Autodesk Inventor part; units mm, degrees
(part 2 of 2)
  measures "d102" distance from line of L722 point (11.407, 32.366)
  measures "d103" distance of point (11.407, 32.366) L722.start
  measures "d104" distance from line of point (37.447, 72.366) L723
  measures "d105" horizontal distance of A1.centre point (49.32, 36.16)
  measures "d106" horizontal distance of point (49.32, 36.16) A1.centre
extrude "Extrusion7" cut sketch "Sketch11" against normal blind 10 contours L0 L1 L2 L3 | L6 L7 L8 L9 | L10 L11 L12 L13 | L14 L15 L16 L17 | L18 L19 L20 L21 | L22 L23 L24 L25 | A0 L365 L362 L363 | A0 L312 L313 L310 L311 | A0 L144 L145 L142 L143 | L62 L63 L64 L65 | L66 L67 L68 L69 | L70 L71 L72 L73 | L74 L75 L76 L77 | L78 L79 L80 L81 | L82 L83 L84 L85 | L122 L123 L124 L125 | L126 L127 L128 L129 | L130 L131 L132 L133 | L134 L135 L136 L137 | L138 L139 L140 L141 | L182 L183 L184 L185 | L186 L187 L188 L189 | L190 L191 L192 L193 | L194 L195 L196 L197 | L198 L199 L200 L201 | L242 L243 L244 L245 | L246 L247 L248 L249 | L250 L251 L252 L253 | L254 L255 L256 L257 | L302 L303 L304 L305 | L306 L307 L308 L309
sketch "Sketch12" plane through (0, 2, 0) normal (0, 1, 0) x (1, 0, 0)
  line L0 (37.4067, 37.3658) -> (39.4067, 37.3658)
  line L1 (39.4067, 37.3658) -> (39.4067, 39.3658)
  line L2 (39.4067, 39.3658) -> (37.4067, 39.3658)
  line L3 (37.4067, 39.3658) -> (37.4067, 37.3658)
  line L4 (35.4067, 37.3658) -> (33.4067, 37.3658) projected
  line L5 (37.4067, 42.8658) -> (39.4067, 42.8658)
  line L6 (39.4067, 42.8658) -> (39.4067, 44.8658)
  line L7 (39.4067, 44.8658) -> (37.4067, 44.8658)
  line L8 (37.4067, 44.8658) -> (37.4067, 42.8658)
  line L9 (37.4067, 48.3658) -> (39.4067, 48.3658)
  line L10 (39.4067, 48.3658) -> (39.4067, 50.3658)
  line L11 (39.4067, 50.3658) -> (37.4067, 50.3658)
  line L12 (37.4067, 50.3658) -> (37.4067, 48.3658)
  line L13 (37.4067, 53.8658) -> (39.4067, 53.8658)
  line L14 (39.4067, 53.8658) -> (39.4067, 55.8658)
  line L15 (39.4067, 55.8658) -> (37.4067, 55.8658)
  line L16 (37.4067, 55.8658) -> (37.4067, 53.8658)
  line L17 (37.4067, 59.3658) -> (39.4067, 59.3658)
  line L18 (39.4067, 59.3658) -> (39.4067, 61.3658)
  line L19 (39.4067, 61.3658) -> (37.4067, 61.3658)
  line L20 (37.4067, 61.3658) -> (37.4067, 59.3658)
  line L21 (37.4067, 64.8658) -> (39.4067, 64.8658)
  line L22 (39.4067, 64.8658) -> (39.4067, 66.8658)
  line L23 (39.4067, 66.8658) -> (37.4067, 66.8658)
  line L24 (37.4067, 66.8658) -> (37.4067, 64.8658)
  line L25 (37.4067, 70.3658) -> (39.4067, 70.3658)
  line L26 (39.4067, 70.3658) -> (39.4067, 72.3658)
  line L27 (39.4067, 72.3658) -> (37.4067, 72.3658)
  line L28 (37.4067, 72.3658) -> (37.4067, 70.3658)
  line L29 (41.4067, 37.3658) -> (43.4067, 37.3658)
  line L30 (43.4067, 37.3658) -> (43.4067, 39.3658)
  line L31 (43.4067, 39.3658) -> (41.4067, 39.3658)
  line L32 (41.4067, 39.3658) -> (41.4067, 37.3658)
  line L33 (41.4067, 42.8658) -> (43.4067, 42.8658)
  line L34 (43.4067, 42.8658) -> (43.4067, 44.8658)
  line L35 (43.4067, 44.8658) -> (41.4067, 44.8658)
  line L36 (41.4067, 44.8658) -> (41.4067, 42.8658)
  line L37 (41.4067, 48.3658) -> (43.4067, 48.3658)
  line L38 (43.4067, 48.3658) -> (43.4067, 50.3658)
  line L39 (43.4067, 50.3658) -> (41.4067, 50.3658)
  line L40 (41.4067, 50.3658) -> (41.4067, 48.3658)
  line L41 (41.4067, 53.8658) -> (43.4067, 53.8658)
  line L42 (43.4067, 53.8658) -> (43.4067, 55.8658)
  line L43 (43.4067, 55.8658) -> (41.4067, 55.8658)
  line L44 (41.4067, 55.8658) -> (41.4067, 53.8658)
  line L45 (41.4067, 59.3658) -> (43.4067, 59.3658)
  line L46 (43.4067, 59.3658) -> (43.4067, 61.3658)
  line L47 (43.4067, 61.3658) -> (41.4067, 61.3658)
  line L48 (41.4067, 61.3658) -> (41.4067, 59.3658)
  line L49 (41.4067, 64.8658) -> (43.4067, 64.8658)
  line L50 (43.4067, 64.8658) -> (43.4067, 66.8658)
  line L51 (43.4067, 66.8658) -> (41.4067, 66.8658)
  line L52 (41.4067, 66.8658) -> (41.4067, 64.8658)
  line L53 (41.4067, 70.3658) -> (43.4067, 70.3658)
  line L54 (43.4067, 70.3658) -> (43.4067, 72.3658)
  line L55 (43.4067, 72.3658) -> (41.4067, 72.3658)
  line L56 (41.4067, 72.3658) -> (41.4067, 70.3658)
  line L57 (45.4067, 37.3658) -> (47.4067, 37.3658)
  line L58 (47.4067, 37.3658) -> (47.4067, 39.3658)
  line L59 (47.4067, 39.3658) -> (45.4067, 39.3658)
  line L60 (45.4067, 39.3658) -> (45.4067, 37.3658)
  line L61 (45.4067, 42.8658) -> (47.4067, 42.8658)
  line L62 (47.4067, 42.8658) -> (47.4067, 44.8658)
  line L63 (47.4067, 44.8658) -> (45.4067, 44.8658)
  line L64 (45.4067, 44.8658) -> (45.4067, 42.8658)
  line L65 (45.4067, 48.3658) -> (47.4067, 48.3658)
  line L66 (47.4067, 48.3658) -> (47.4067, 50.3658)
  line L67 (47.4067, 50.3658) -> (45.4067, 50.3658)
  line L68 (45.4067, 50.3658) -> (45.4067, 48.3658)
  line L69 (45.4067, 53.8658) -> (47.4067, 53.8658)
  line L70 (47.4067, 53.8658) -> (47.4067, 55.8658)
  line L71 (47.4067, 55.8658) -> (45.4067, 55.8658)
  line L72 (45.4067, 55.8658) -> (45.4067, 53.8658)
  line L73 (45.4067, 59.3658) -> (47.4067, 59.3658)
  line L74 (47.4067, 59.3658) -> (47.4067, 61.3658)
  line L75 (47.4067, 61.3658) -> (45.4067, 61.3658)
  line L76 (45.4067, 61.3658) -> (45.4067, 59.3658)
  line L77 (45.4067, 64.8658) -> (47.4067, 64.8658)
  line L78 (47.4067, 64.8658) -> (47.4067, 66.8658)
  line L79 (47.4067, 66.8658) -> (45.4067, 66.8658)
  line L80 (45.4067, 66.8658) -> (45.4067, 64.8658)
  line L81 (45.4067, 70.3658) -> (47.4067, 70.3658)
  line L82 (47.4067, 70.3658) -> (47.4067, 72.3658)
  line L83 (47.4067, 72.3658) -> (45.4067, 72.3658)
  line L84 (45.4067, 72.3658) -> (45.4067, 70.3658)
  line L85 (49.4067, 37.3658) -> (51.4067, 37.3658)
  line L86 (51.4067, 37.3658) -> (51.4067, 39.3658)
  line L87 (51.4067, 39.3658) -> (49.4067, 39.3658)
  line L88 (49.4067, 39.3658) -> (49.4067, 37.3658)
  line L89 (49.4067, 42.8658) -> (51.4067, 42.8658)
  line L90 (51.4067, 42.8658) -> (51.4067, 44.8658)
  line L91 (51.4067, 44.8658) -> (49.4067, 44.8658)
  line L92 (49.4067, 44.8658) -> (49.4067, 42.8658)
  line L93 (49.4067, 48.3658) -> (51.4067, 48.3658)
  line L94 (51.4067, 48.3658) -> (51.4067, 50.3658)
  line L95 (51.4067, 50.3658) -> (49.4067, 50.3658)
  line L96 (49.4067, 50.3658) -> (49.4067, 48.3658)
  line L97 (49.4067, 53.8658) -> (51.4067, 53.8658)
  line L98 (51.4067, 53.8658) -> (51.4067, 55.8658)
  line L99 (51.4067, 55.8658) -> (49.4067, 55.8658)
  line L100 (49.4067, 55.8658) -> (49.4067, 53.8658)
  line L101 (49.4067, 59.3658) -> (51.4067, 59.3658)
  line L102 (51.4067, 59.3658) -> (51.4067, 61.3658)
  line L103 (51.4067, 61.3658) -> (49.4067, 61.3658)
  line L104 (49.4067, 61.3658) -> (49.4067, 59.3658)
  line L105 (49.4067, 64.8658) -> (51.4067, 64.8658)
  line L106 (51.4067, 64.8658) -> (51.4067, 66.8658)
  line L107 (51.4067, 66.8658) -> (49.4067, 66.8658)
  line L108 (49.4067, 66.8658) -> (49.4067, 64.8658)
  line L109 (49.4067, 70.3658) -> (51.4067, 70.3658)
  line L110 (51.4067, 70.3658) -> (51.4067, 72.3658)
  line L111 (51.4067, 72.3658) -> (49.4067, 72.3658)
  line L112 (49.4067, 72.3658) -> (49.4067, 70.3658)
  line L113 (53.4067, 37.3658) -> (55.4067, 37.3658)
  line L114 (55.4067, 37.3658) -> (55.4067, 39.3658)
  line L115 (55.4067, 39.3658) -> (53.4067, 39.3658)
  line L116 (53.4067, 39.3658) -> (53.4067, 37.3658)
  line L117 (53.4067, 42.8658) -> (55.4067, 42.8658)
  line L118 (55.4067, 42.8658) -> (55.4067, 44.8658)
  line L119 (55.4067, 44.8658) -> (53.4067, 44.8658)
  line L120 (53.4067, 44.8658) -> (53.4067, 42.8658)
  line L121 (53.4067, 48.3658) -> (55.4067, 48.3658)
  line L122 (55.4067, 48.3658) -> (55.4067, 50.3658)
  line L123 (55.4067, 50.3658) -> (53.4067, 50.3658)
  line L124 (53.4067, 50.3658) -> (53.4067, 48.3658)
  line L125 (53.4067, 53.8658) -> (55.4067, 53.8658)
  line L126 (55.4067, 53.8658) -> (55.4067, 55.8658)
  line L127 (55.4067, 55.8658) -> (53.4067, 55.8658)
  line L128 (53.4067, 55.8658) -> (53.4067, 53.8658)
  line L129 (53.4067, 59.3658) -> (55.4067, 59.3658)
  line L130 (55.4067, 59.3658) -> (55.4067, 61.3658)
  line L131 (55.4067, 61.3658) -> (53.4067, 61.3658)
  line L132 (53.4067, 61.3658) -> (53.4067, 59.3658)
  line L133 (53.4067, 64.8658) -> (55.4067, 64.8658)
  line L134 (55.4067, 64.8658) -> (55.4067, 66.8658)
  line L135 (55.4067, 66.8658) -> (53.4067, 66.8658)
  line L136 (53.4067, 66.8658) -> (53.4067, 64.8658)
  line L137 (53.4067, 70.3658) -> (55.4067, 70.3658)
  line L138 (55.4067, 70.3658) -> (55.4067, 72.3658)
  line L139 (55.4067, 72.3658) -> (53.4067, 72.3658)
  line L140 (53.4067, 72.3658) -> (53.4067, 70.3658)
  line L141 (57.4067, 37.3658) -> (59.4067, 37.3658)
  line L142 (59.4067, 37.3658) -> (59.4067, 39.3658)
  line L143 (59.4067, 39.3658) -> (57.4067, 39.3658)
  line L144 (57.4067, 39.3658) -> (57.4067, 37.3658)
  line L145 (57.4067, 42.8658) -> (59.4067, 42.8658)
  line L146 (59.4067, 42.8658) -> (59.4067, 44.8658)
  line L147 (59.4067, 44.8658) -> (57.4067, 44.8658)
  line L148 (57.4067, 44.8658) -> (57.4067, 42.8658)
  line L149 (57.4067, 48.3658) -> (59.4067, 48.3658)
  line L150 (59.4067, 48.3658) -> (59.4067, 50.3658)
  line L151 (59.4067, 50.3658) -> (57.4067, 50.3658)
  line L152 (57.4067, 50.3658) -> (57.4067, 48.3658)
  line L153 (57.4067, 53.8658) -> (59.4067, 53.8658)
  line L154 (59.4067, 53.8658) -> (59.4067, 55.8658)
  line L155 (59.4067, 55.8658) -> (57.4067, 55.8658)
  line L156 (57.4067, 55.8658) -> (57.4067, 53.8658)
  line L157 (57.4067, 59.3658) -> (59.4067, 59.3658)
  line L158 (59.4067, 59.3658) -> (59.4067, 61.3658)
  line L159 (59.4067, 61.3658) -> (57.4067, 61.3658)
  line L160 (57.4067, 61.3658) -> (57.4067, 59.3658)
  line L161 (57.4067, 64.8658) -> (59.4067, 64.8658)
  line L162 (59.4067, 64.8658) -> (59.4067, 66.8658)
  line L163 (59.4067, 66.8658) -> (57.4067, 66.8658)
  line L164 (57.4067, 66.8658) -> (57.4067, 64.8658)
  line L165 (57.4067, 70.3658) -> (59.4067, 70.3658)
  line L166 (59.4067, 70.3658) -> (59.4067, 72.3658)
  line L167 (59.4067, 72.3658) -> (57.4067, 72.3658)
  line L168 (57.4067, 72.3658) -> (57.4067, 70.3658)
  line L169 (61.4067, 37.3658) -> (63.4067, 37.3658)
  line L170 (63.4067, 37.3658) -> (63.4067, 39.3658)
  line L171 (63.4067, 39.3658) -> (61.4067, 39.3658)
  line L172 (61.4067, 39.3658) -> (61.4067, 37.3658)
  line L173 (61.4067, 42.8658) -> (63.4067, 42.8658)
  line L174 (63.4067, 42.8658) -> (63.4067, 44.8658)
  line L175 (63.4067, 44.8658) -> (61.4067, 44.8658)
  line L176 (61.4067, 44.8658) -> (61.4067, 42.8658)
  line L177 (61.4067, 48.3658) -> (63.4067, 48.3658)
  line L178 (63.4067, 48.3658) -> (63.4067, 50.3658)
  line L179 (63.4067, 50.3658) -> (61.4067, 50.3658)
  line L180 (61.4067, 50.3658) -> (61.4067, 48.3658)
  line L181 (61.4067, 53.8658) -> (63.4067, 53.8658)
  line L182 (63.4067, 53.8658) -> (63.4067, 55.8658)
  line L183 (63.4067, 55.8658) -> (61.4067, 55.8658)
  line L184 (61.4067, 55.8658) -> (61.4067, 53.8658)
  line L185 (61.4067, 59.3658) -> (63.4067, 59.3658)
  line L186 (63.4067, 59.3658) -> (63.4067, 61.3658)
  line L187 (63.4067, 61.3658) -> (61.4067, 61.3658)
  line L188 (61.4067, 61.3658) -> (61.4067, 59.3658)
  line L189 (61.4067, 64.8658) -> (63.4067, 64.8658)
  line L190 (63.4067, 64.8658) -> (63.4067, 66.8658)
  line L191 (63.4067, 66.8658) -> (61.4067, 66.8658)
  line L192 (61.4067, 66.8658) -> (61.4067, 64.8658)
  line L193 (61.4067, 70.3658) -> (63.4067, 70.3658)
  line L194 (63.4067, 70.3658) -> (63.4067, 72.3658)
  line L195 (63.4067, 72.3658) -> (61.4067, 72.3658)
  line L196 (61.4067, 72.3658) -> (61.4067, 70.3658)
  line L197 (65.4067, 37.3658) -> (67.4067, 37.3658)
  line L198 (67.4067, 37.3658) -> (67.4067, 39.3658)
  line L199 (67.4067, 39.3658) -> (65.4067, 39.3658)
  line L200 (65.4067, 39.3658) -> (65.4067, 37.3658)
  line L201 (65.4067, 42.8658) -> (67.4067, 42.8658)
  line L202 (67.4067, 42.8658) -> (67.4067, 44.8658)
  line L203 (67.4067, 44.8658) -> (65.4067, 44.8658)
  line L204 (65.4067, 44.8658) -> (65.4067, 42.8658)
  line L205 (65.4067, 48.3658) -> (67.4067, 48.3658)
  line L206 (67.4067, 48.3658) -> (67.4067, 50.3658)
  line L207 (67.4067, 50.3658) -> (65.4067, 50.3658)
  line L208 (65.4067, 50.3658) -> (65.4067, 48.3658)
  line L209 (65.4067, 53.8658) -> (67.4067, 53.8658)
  line L210 (67.4067, 53.8658) -> (67.4067, 55.8658)
  line L211 (67.4067, 55.8658) -> (65.4067, 55.8658)
  line L212 (65.4067, 55.8658) -> (65.4067, 53.8658)
  line L213 (65.4067, 59.3658) -> (67.4067, 59.3658)
  line L214 (67.4067, 59.3658) -> (67.4067, 61.3658)
  line L215 (67.4067, 61.3658) -> (65.4067, 61.3658)
  line L216 (65.4067, 61.3658) -> (65.4067, 59.3658)
  line L217 (65.4067, 64.8658) -> (67.4067, 64.8658)
  line L218 (67.4067, 64.8658) -> (67.4067, 66.8658)
  line L219 (67.4067, 66.8658) -> (65.4067, 66.8658)
  line L220 (65.4067, 66.8658) -> (65.4067, 64.8658)
  line L221 (65.4067, 70.3658) -> (67.4067, 70.3658)
  line L222 (67.4067, 70.3658) -> (67.4067, 72.3658)
  line L223 (67.4067, 72.3658) -> (65.4067, 72.3658)
  line L224 (65.4067, 72.3658) -> (65.4067, 70.3658)
  line L225 (69.4067, 37.3658) -> (71.4067, 37.3658)
  line L226 (71.4067, 37.3658) -> (71.4067, 39.3658)
  line L227 (71.4067, 39.3658) -> (69.4067, 39.3658)
  line L228 (69.4067, 39.3658) -> (69.4067, 37.3658)
  line L229 (69.4067, 42.8658) -> (71.4067, 42.8658)
  line L230 (71.4067, 42.8658) -> (71.4067, 44.8658)
  line L231 (71.4067, 44.8658) -> (69.4067, 44.8658)
  line L232 (69.4067, 44.8658) -> (69.4067, 42.8658)
  line L233 (69.4067, 48.3658) -> (71.4067, 48.3658)
  line L234 (71.4067, 48.3658) -> (71.4067, 50.3658)
  line L235 (71.4067, 50.3658) -> (69.4067, 50.3658)
  line L236 (69.4067, 50.3658) -> (69.4067, 48.3658)
  line L237 (69.4067, 53.8658) -> (71.4067, 53.8658)
  line L238 (71.4067, 53.8658) -> (71.4067, 55.8658)
  line L239 (71.4067, 55.8658) -> (69.4067, 55.8658)
  line L240 (69.4067, 55.8658) -> (69.4067, 53.8658)
  line L241 (69.4067, 59.3658) -> (71.4067, 59.3658)
  line L242 (71.4067, 59.3658) -> (71.4067, 61.3658)
  line L243 (71.4067, 61.3658) -> (69.4067, 61.3658)
  line L244 (69.4067, 61.3658) -> (69.4067, 59.3658)
  line L245 (69.4067, 64.8658) -> (71.4067, 64.8658)
  line L246 (71.4067, 64.8658) -> (71.4067, 66.8658)
  line L247 (71.4067, 66.8658) -> (69.4067, 66.8658)
  line L248 (69.4067, 66.8658) -> (69.4067, 64.8658)
  line L249 (69.4067, 70.3658) -> (71.4067, 70.3658)
  line L250 (71.4067, 70.3658) -> (71.4067, 72.3658)
  line L251 (71.4067, 72.3658) -> (69.4067, 72.3658)
  line L252 (69.4067, 72.3658) -> (69.4067, 70.3658)
  line L253 (73.4067, 37.3658) -> (75.4067, 37.3658)
  line L254 (75.4067, 37.3658) -> (75.4067, 39.3658)
  line L255 (75.4067, 39.3658) -> (73.4067, 39.3658)
  line L256 (73.4067, 39.3658) -> (73.4067, 37.3658)
  line L257 (73.4067, 42.8658) -> (75.4067, 42.8658)
  line L258 (75.4067, 42.8658) -> (75.4067, 44.8658)
  line L259 (75.4067, 44.8658) -> (73.4067, 44.8658)
  line L260 (73.4067, 44.8658) -> (73.4067, 42.8658)
  line L261 (73.4067, 48.3658) -> (75.4067, 48.3658)
  line L262 (75.4067, 48.3658) -> (75.4067, 50.3658)
  line L263 (75.4067, 50.3658) -> (73.4067, 50.3658)
  line L264 (73.4067, 50.3658) -> (73.4067, 48.3658)
  line L265 (73.4067, 53.8658) -> (75.4067, 53.8658)
  line L266 (75.4067, 53.8658) -> (75.4067, 55.8658)
  line L267 (75.4067, 55.8658) -> (73.4067, 55.8658)
  line L268 (73.4067, 55.8658) -> (73.4067, 53.8658)
  line L269 (73.4067, 59.3658) -> (75.4067, 59.3658)
  line L270 (75.4067, 59.3658) -> (75.4067, 61.3658)
  line L271 (75.4067, 61.3658) -> (73.4067, 61.3658)
  line L272 (73.4067, 61.3658) -> (73.4067, 59.3658)
  line L273 (73.4067, 64.8658) -> (75.4067, 64.8658)
  line L274 (75.4067, 64.8658) -> (75.4067, 66.8658)
  line L275 (75.4067, 66.8658) -> (73.4067, 66.8658)
  line L276 (73.4067, 66.8658) -> (73.4067, 64.8658)
  line L277 (73.4067, 70.3658) -> (75.4067, 70.3658)
  line L278 (75.4067, 70.3658) -> (75.4067, 72.3658)
  line L279 (75.4067, 72.3658) -> (73.4067, 72.3658)
  line L280 (73.4067, 72.3658) -> (73.4067, 70.3658)
  line L281 (77.4067, 37.3658) -> (79.4067, 37.3658)
  line L282 (79.4067, 37.3658) -> (79.4067, 39.3658)
  line L283 (79.4067, 39.3658) -> (77.4067, 39.3658)
  line L284 (77.4067, 39.3658) -> (77.4067, 37.3658)
  line L285 (77.4067, 42.8658) -> (79.4067, 42.8658)
  line L286 (79.4067, 42.8658) -> (79.4067, 44.8658)
  line L287 (79.4067, 44.8658) -> (77.4067, 44.8658)
  line L288 (77.4067, 44.8658) -> (77.4067, 42.8658)
  line L289 (77.4067, 48.3658) -> (79.4067, 48.3658)
  line L290 (79.4067, 48.3658) -> (79.4067, 50.3658)
  line L291 (79.4067, 50.3658) -> (77.4067, 50.3658)
  line L292 (77.4067, 50.3658) -> (77.4067, 48.3658)
  line L293 (77.4067, 53.8658) -> (79.4067, 53.8658)
  line L294 (79.4067, 53.8658) -> (79.4067, 55.8658)
  line L295 (79.4067, 55.8658) -> (77.4067, 55.8658)
  line L296 (77.4067, 55.8658) -> (77.4067, 53.8658)
  line L297 (77.4067, 59.3658) -> (79.4067, 59.3658)
  line L298 (79.4067, 59.3658) -> (79.4067, 61.3658)
  line L299 (79.4067, 61.3658) -> (77.4067, 61.3658)
  line L300 (77.4067, 61.3658) -> (77.4067, 59.3658)
  line L301 (77.4067, 64.8658) -> (79.4067, 64.8658)
  line L302 (79.4067, 64.8658) -> (79.4067, 66.8658)
  line L303 (79.4067, 66.8658) -> (77.4067, 66.8658)
  line L304 (77.4067, 66.8658) -> (77.4067, 64.8658)
  line L305 (77.4067, 70.3658) -> (79.4067, 70.3658)
  line L306 (79.4067, 70.3658) -> (79.4067, 72.3658)
  line L307 (79.4067, 72.3658) -> (77.4067, 72.3658)
  line L308 (77.4067, 72.3658) -> (77.4067, 70.3658)
  line L309 (81.4067, 37.3658) -> (83.4067, 37.3658)
  line L310 (83.4067, 37.3658) -> (83.4067, 39.3658)
  line L311 (83.4067, 39.3658) -> (81.4067, 39.3658)
  line L312 (81.4067, 39.3658) -> (81.4067, 37.3658)
  line L313 (81.4067, 42.8658) -> (83.4067, 42.8658)
  line L314 (83.4067, 42.8658) -> (83.4067, 44.8658)
  line L315 (83.4067, 44.8658) -> (81.4067, 44.8658)
  line L316 (81.4067, 44.8658) -> (81.4067, 42.8658)
  line L317 (81.4067, 48.3658) -> (83.4067, 48.3658)
  line L318 (83.4067, 48.3658) -> (83.4067, 50.3658)
  line L319 (83.4067, 50.3658) -> (81.4067, 50.3658)
  line L320 (81.4067, 50.3658) -> (81.4067, 48.3658)
  line L321 (81.4067, 53.8658) -> (83.4067, 53.8658)
  line L322 (83.4067, 53.8658) -> (83.4067, 55.8658)
  line L323 (83.4067, 55.8658) -> (81.4067, 55.8658)
  line L324 (81.4067, 55.8658) -> (81.4067, 53.8658)
  line L325 (81.4067, 59.3658) -> (83.4067, 59.3658)
  line L326 (83.4067, 59.3658) -> (83.4067, 61.3658)
  line L327 (83.4067, 61.3658) -> (81.4067, 61.3658)
  line L328 (81.4067, 61.3658) -> (81.4067, 59.3658)
  line L329 (81.4067, 64.8658) -> (83.4067, 64.8658)
  line L330 (83.4067, 64.8658) -> (83.4067, 66.8658)
  line L331 (83.4067, 66.8658) -> (81.4067, 66.8658)
  line L332 (81.4067, 66.8658) -> (81.4067, 64.8658)
  line L333 (81.4067, 70.3658) -> (83.4067, 70.3658)
  line L334 (83.4067, 70.3658) -> (83.4067, 72.3658)
  line L335 (83.4067, 72.3658) -> (81.4067, 72.3658)
  line L336 (81.4067, 72.3658) -> (81.4067, 70.3658)
  line L337 (85.4067, 37.3658) -> (87.4067, 37.3658)
  line L338 (87.4067, 37.3658) -> (87.4067, 39.3658)
  line L339 (87.4067, 39.3658) -> (85.4067, 39.3658)
  line L340 (85.4067, 39.3658) -> (85.4067, 37.3658)
  line L341 (85.4067, 42.8658) -> (87.4067, 42.8658)
  line L342 (87.4067, 42.8658) -> (87.4067, 44.8658)
  line L343 (87.4067, 44.8658) -> (85.4067, 44.8658)
  line L344 (85.4067, 44.8658) -> (85.4067, 42.8658)
  line L345 (85.4067, 48.3658) -> (87.4067, 48.3658)
  line L346 (87.4067, 48.3658) -> (87.4067, 50.3658)
  line L347 (87.4067, 50.3658) -> (85.4067, 50.3658)
  line L348 (85.4067, 50.3658) -> (85.4067, 48.3658)
  line L349 (85.4067, 53.8658) -> (87.4067, 53.8658)
  line L350 (87.4067, 53.8658) -> (87.4067, 55.8658)
  line L351 (87.4067, 55.8658) -> (85.4067, 55.8658)
  line L352 (85.4067, 55.8658) -> (85.4067, 53.8658)
  line L353 (85.4067, 59.3658) -> (87.4067, 59.3658)
  line L354 (87.4067, 59.3658) -> (87.4067, 61.3658)
  line L355 (87.4067, 61.3658) -> (85.4067, 61.3658)
  line L356 (85.4067, 61.3658) -> (85.4067, 59.3658)
  line L357 (85.4067, 64.8658) -> (87.4067, 64.8658)
  line L358 (87.4067, 64.8658) -> (87.4067, 66.8658)
  line L359 (87.4067, 66.8658) -> (85.4067, 66.8658)
  line L360 (85.4067, 66.8658) -> (85.4067, 64.8658)
  line L361 (85.4067, 70.3658) -> (87.4067, 70.3658)
  line L362 (87.4067, 70.3658) -> (87.4067, 72.3658)
  line L363 (87.4067, 72.3658) -> (85.4067, 72.3658)
  line L364 (85.4067, 72.3658) -> (85.4067, 70.3658)
  line L365 (89.4067, 37.3658) -> (91.4067, 37.3658)
  line L366 (91.4067, 37.3658) -> (91.4067, 39.3658)
  line L367 (91.4067, 39.3658) -> (89.4067, 39.3658)
  line L368 (89.4067, 39.3658) -> (89.4067, 37.3658)
  line L369 (89.4067, 42.8658) -> (91.4067, 42.8658)
  line L370 (91.4067, 42.8658) -> (91.4067, 44.8658)
  line L371 (91.4067, 44.8658) -> (89.4067, 44.8658)
  line L372 (89.4067, 44.8658) -> (89.4067, 42.8658)
  line L373 (89.4067, 48.3658) -> (91.4067, 48.3658)
  line L374 (91.4067, 48.3658) -> (91.4067, 50.3658)
  line L375 (91.4067, 50.3658) -> (89.4067, 50.3658)
  line L376 (89.4067, 50.3658) -> (89.4067, 48.3658)
  line L377 (89.4067, 53.8658) -> (91.4067, 53.8658)
  line L378 (91.4067, 53.8658) -> (91.4067, 55.8658)
  line L379 (91.4067, 55.8658) -> (89.4067, 55.8658)
  line L380 (89.4067, 55.8658) -> (89.4067, 53.8658)
  line L381 (89.4067, 59.3658) -> (91.4067, 59.3658)
  line L382 (91.4067, 59.3658) -> (91.4067, 61.3658)
  line L383 (91.4067, 61.3658) -> (89.4067, 61.3658)
  line L384 (89.4067, 61.3658) -> (89.4067, 59.3658)
  line L385 (89.4067, 64.8658) -> (91.4067, 64.8658)
  line L386 (91.4067, 64.8658) -> (91.4067, 66.8658)
  line L387 (91.4067, 66.8658) -> (89.4067, 66.8658)
  line L388 (89.4067, 66.8658) -> (89.4067, 64.8658)
  line L389 (89.4067, 70.3658) -> (91.4067, 70.3658)
  line L390 (91.4067, 70.3658) -> (91.4067, 72.3658)
  line L391 (91.4067, 72.3658) -> (89.4067, 72.3658)
  line L392 (89.4067, 72.3658) -> (89.4067, 70.3658)
  line L393 (93.4067, 37.3658) -> (95.4067, 37.3658)
  line L394 (95.4067, 37.3658) -> (95.4067, 39.3658)
  line L395 (95.4067, 39.3658) -> (93.4067, 39.3658)
  line L396 (93.4067, 39.3658) -> (93.4067, 37.3658)
  line L397 (93.4067, 42.8658) -> (95.4067, 42.8658)
  line L398 (95.4067, 42.8658) -> (95.4067, 44.8658)
  line L399 (95.4067, 44.8658) -> (93.4067, 44.8658)
  line L400 (93.4067, 44.8658) -> (93.4067, 42.8658)
  line L401 (93.4067, 48.3658) -> (95.4067, 48.3658)
  line L402 (95.4067, 48.3658) -> (95.4067, 50.3658)
  line L403 (95.4067, 50.3658) -> (93.4067, 50.3658)
  line L404 (93.4067, 50.3658) -> (93.4067, 48.3658)
  line L405 (93.4067, 53.8658) -> (95.4067, 53.8658)
  line L406 (95.4067, 53.8658) -> (95.4067, 55.8658)
  line L407 (95.4067, 55.8658) -> (93.4067, 55.8658)
  line L408 (93.4067, 55.8658) -> (93.4067, 53.8658)
  line L409 (93.4067, 59.3658) -> (95.4067, 59.3658)
  line L410 (95.4067, 59.3658) -> (95.4067, 61.3658)
  line L411 (95.4067, 61.3658) -> (93.4067, 61.3658)
  line L412 (93.4067, 61.3658) -> (93.4067, 59.3658)
  line L413 (93.4067, 64.8658) -> (95.4067, 64.8658)
  line L414 (95.4067, 64.8658) -> (95.4067, 66.8658)
  line L415 (95.4067, 66.8658) -> (93.4067, 66.8658)
  line L416 (93.4067, 66.8658) -> (93.4067, 64.8658)
  line L417 (93.4067, 70.3658) -> (95.4067, 70.3658)
  line L418 (95.4067, 70.3658) -> (95.4067, 72.3658)
  line L419 (95.4067, 72.3658) -> (93.4067, 72.3658)
  line L420 (93.4067, 72.3658) -> (93.4067, 70.3658)
  line L421 (97.4067, 37.3658) -> (99.4067, 37.3658)
  line L422 (99.4067, 37.3658) -> (99.4067, 39.3658)
  line L423 (99.4067, 39.3658) -> (97.4067, 39.3658)
  line L424 (97.4067, 39.3658) -> (97.4067, 37.3658)
  line L425 (97.4067, 42.8658) -> (99.4067, 42.8658)
  line L426 (99.4067, 42.8658) -> (99.4067, 44.8658)
  line L427 (99.4067, 44.8658) -> (97.4067, 44.8658)
  line L428 (97.4067, 44.8658) -> (97.4067, 42.8658)
  line L429 (97.4067, 48.3658) -> (99.4067, 48.3658)
  line L430 (99.4067, 48.3658) -> (99.4067, 50.3658)
  line L431 (99.4067, 50.3658) -> (97.4067, 50.3658)
  line L432 (97.4067, 50.3658) -> (97.4067, 48.3658)
  line L433 (97.4067, 53.8658) -> (99.4067, 53.8658)
  line L434 (99.4067, 53.8658) -> (99.4067, 55.8658)
  line L435 (99.4067, 55.8658) -> (97.4067, 55.8658)
  line L436 (97.4067, 55.8658) -> (97.4067, 53.8658)
  line L437 (97.4067, 59.3658) -> (99.4067, 59.3658)
  line L438 (99.4067, 59.3658) -> (99.4067, 61.3658)
  line L439 (99.4067, 61.3658) -> (97.4067, 61.3658)
  line L440 (97.4067, 61.3658) -> (97.4067, 59.3658)
  line L441 (97.4067, 64.8658) -> (99.4067, 64.8658)
  line L442 (99.4067, 64.8658) -> (99.4067, 66.8658)
  line L443 (99.4067, 66.8658) -> (97.4067, 66.8658)
  line L444 (97.4067, 66.8658) -> (97.4067, 64.8658)
  line L445 (97.4067, 70.3658) -> (99.4067, 70.3658)
  line L446 (99.4067, 70.3658) -> (99.4067, 72.3658)
  line L447 (99.4067, 72.3658) -> (97.4067, 72.3658)
  line L448 (97.4067, 72.3658) -> (97.4067, 70.3658)
  line L449 (101.4067, 37.3658) -> (103.4067, 37.3658)
  line L450 (103.4067, 37.3658) -> (103.4067, 39.3658)
  line L451 (103.4067, 39.3658) -> (101.4067, 39.3658)
  line L452 (101.4067, 39.3658) -> (101.4067, 37.3658)
  line L453 (101.4067, 42.8658) -> (103.4067, 42.8658)
  line L454 (103.4067, 42.8658) -> (103.4067, 44.8658)
  line L455 (103.4067, 44.8658) -> (101.4067, 44.8658)
  line L456 (101.4067, 44.8658) -> (101.4067, 42.8658)
  line L457 (101.4067, 48.3658) -> (103.4067, 48.3658)
  line L458 (103.4067, 48.3658) -> (103.4067, 50.3658)
  line L459 (103.4067, 50.3658) -> (101.4067, 50.3658)
  line L460 (101.4067, 50.3658) -> (101.4067, 48.3658)
  line L461 (101.4067, 53.8658) -> (103.4067, 53.8658)
  line L462 (103.4067, 53.8658) -> (103.4067, 55.8658)
  line L463 (103.4067, 55.8658) -> (101.4067, 55.8658)
  line L464 (101.4067, 55.8658) -> (101.4067, 53.8658)
  line L465 (101.4067, 59.3658) -> (103.4067, 59.3658)
  line L466 (103.4067, 59.3658) -> (103.4067, 61.3658)
  line L467 (103.4067, 61.3658) -> (101.4067, 61.3658)
  line L468 (101.4067, 61.3658) -> (101.4067, 59.3658)
  line L469 (101.4067, 64.8658) -> (103.4067, 64.8658)
  line L470 (103.4067, 64.8658) -> (103.4067, 66.8658)
  line L471 (103.4067, 66.8658) -> (101.4067, 66.8658)
  line L472 (101.4067, 66.8658) -> (101.4067, 64.8658)
  line L473 (101.4067, 70.3658) -> (103.4067, 70.3658)
  line L474 (103.4067, 70.3658) -> (103.4067, 72.3658)
  line L475 (103.4067, 72.3658) -> (101.4067, 72.3658)
  line L476 (101.4067, 72.3658) -> (101.4067, 70.3658)
  line L477 (105.4067, 37.3658) -> (107.4067, 37.3658)
  line L478 (107.4067, 37.3658) -> (107.4067, 39.3658)
  line L479 (107.4067, 39.3658) -> (105.4067, 39.3658)
  line L480 (105.4067, 39.3658) -> (105.4067, 37.3658)
  line L481 (105.4067, 42.8658) -> (107.4067, 42.8658)
  line L482 (107.4067, 42.8658) -> (107.4067, 44.8658)
  line L483 (107.4067, 44.8658) -> (105.4067, 44.8658)
  line L484 (105.4067, 44.8658) -> (105.4067, 42.8658)
  line L485 (105.4067, 48.3658) -> (107.4067, 48.3658)
  line L486 (107.4067, 48.3658) -> (107.4067, 50.3658)
  line L487 (107.4067, 50.3658) -> (105.4067, 50.3658)
  line L488 (105.4067, 50.3658) -> (105.4067, 48.3658)
  line L489 (105.4067, 53.8658) -> (107.4067, 53.8658)
  line L490 (107.4067, 53.8658) -> (107.4067, 55.8658)
  line L491 (107.4067, 55.8658) -> (105.4067, 55.8658)
  line L492 (105.4067, 55.8658) -> (105.4067, 53.8658)
  line L493 (105.4067, 59.3658) -> (107.4067, 59.3658)
  line L494 (107.4067, 59.3658) -> (107.4067, 61.3658)
  line L495 (107.4067, 61.3658) -> (105.4067, 61.3658)
  line L496 (105.4067, 61.3658) -> (105.4067, 59.3658)
  line L497 (105.4067, 64.8658) -> (107.4067, 64.8658)
  line L498 (107.4067, 64.8658) -> (107.4067, 66.8658)
  line L499 (107.4067, 66.8658) -> (105.4067, 66.8658)
  line L500 (105.4067, 66.8658) -> (105.4067, 64.8658)
  line L501 (105.4067, 70.3658) -> (107.4067, 70.3658)
  line L502 (107.4067, 70.3658) -> (107.4067, 72.3658)
  line L503 (107.4067, 72.3658) -> (105.4067, 72.3658)
  line L504 (105.4067, 72.3658) -> (105.4067, 70.3658)
  line L505 (109.4067, 37.3658) -> (111.4067, 37.3658)
  line L506 (111.4067, 37.3658) -> (111.4067, 39.3658)
  line L507 (111.4067, 39.3658) -> (109.4067, 39.3658)
  line L508 (109.4067, 39.3658) -> (109.4067, 37.3658)
  line L509 (109.4067, 42.8658) -> (111.4067, 42.8658)
  line L510 (111.4067, 42.8658) -> (111.4067, 44.8658)
  line L511 (111.4067, 44.8658) -> (109.4067, 44.8658)
  line L512 (109.4067, 44.8658) -> (109.4067, 42.8658)
  line L513 (109.4067, 48.3658) -> (111.4067, 48.3658)
  line L514 (111.4067, 48.3658) -> (111.4067, 50.3658)
  line L515 (111.4067, 50.3658) -> (109.4067, 50.3658)
  line L516 (109.4067, 50.3658) -> (109.4067, 48.3658)
  line L517 (109.4067, 53.8658) -> (111.4067, 53.8658)
  line L518 (111.4067, 53.8658) -> (111.4067, 55.8658)
  line L519 (111.4067, 55.8658) -> (109.4067, 55.8658)
  line L520 (109.4067, 55.8658) -> (109.4067, 53.8658)
  line L521 (109.4067, 59.3658) -> (111.4067, 59.3658)
  line L522 (111.4067, 59.3658) -> (111.4067, 61.3658)
  line L523 (111.4067, 61.3658) -> (109.4067, 61.3658)
  line L524 (109.4067, 61.3658) -> (109.4067, 59.3658)
  line L525 (109.4067, 64.8658) -> (111.4067, 64.8658)
  line L526 (111.4067, 64.8658) -> (111.4067, 66.8658)
  line L527 (111.4067, 66.8658) -> (109.4067, 66.8658)
  line L528 (109.4067, 66.8658) -> (109.4067, 64.8658)
  line L529 (109.4067, 70.3658) -> (111.4067, 70.3658)
  line L530 (111.4067, 70.3658) -> (111.4067, 72.3658)
  line L531 (111.4067, 72.3658) -> (109.4067, 72.3658)
  line L532 (109.4067, 72.3658) -> (109.4067, 70.3658)
  line L533 (113.4067, 37.3658) -> (115.4067, 37.3658)
  line L534 (115.4067, 37.3658) -> (115.4067, 39.3658)
  line L535 (115.4067, 39.3658) -> (113.4067, 39.3658)
  line L536 (113.4067, 39.3658) -> (113.4067, 37.3658)
  line L537 (113.4067, 42.8658) -> (115.4067, 42.8658)
  line L538 (115.4067, 42.8658) -> (115.4067, 44.8658)
  line L539 (115.4067, 44.8658) -> (113.4067, 44.8658)
  line L540 (113.4067, 44.8658) -> (113.4067, 42.8658)
  line L541 (113.4067, 48.3658) -> (115.4067, 48.3658)
  line L542 (115.4067, 48.3658) -> (115.4067, 50.3658)
  line L543 (115.4067, 50.3658) -> (113.4067, 50.3658)
  line L544 (113.4067, 50.3658) -> (113.4067, 48.3658)
  line L545 (113.4067, 53.8658) -> (115.4067, 53.8658)
  line L546 (115.4067, 53.8658) -> (115.4067, 55.8658)
  line L547 (115.4067, 55.8658) -> (113.4067, 55.8658)
  line L548 (113.4067, 55.8658) -> (113.4067, 53.8658)
  line L549 (113.4067, 59.3658) -> (115.4067, 59.3658)
  line L550 (115.4067, 59.3658) -> (115.4067, 61.3658)
  line L551 (115.4067, 61.3658) -> (113.4067, 61.3658)
  line L552 (113.4067, 61.3658) -> (113.4067, 59.3658)
  line L553 (113.4067, 64.8658) -> (115.4067, 64.8658)
  line L554 (115.4067, 64.8658) -> (115.4067, 66.8658)
  line L555 (115.4067, 66.8658) -> (113.4067, 66.8658)
  line L556 (113.4067, 66.8658) -> (113.4067, 64.8658)
  line L557 (113.4067, 70.3658) -> (115.4067, 70.3658)
  line L558 (115.4067, 70.3658) -> (115.4067, 72.3658)
  line L559 (115.4067, 72.3658) -> (113.4067, 72.3658)
  line L560 (113.4067, 72.3658) -> (113.4067, 70.3658)
  line L561 (117.4067, 37.3658) -> (119.4067, 37.3658)
  line L562 (119.4067, 37.3658) -> (119.4067, 39.3658)
  line L563 (119.4067, 39.3658) -> (117.4067, 39.3658)
  line L564 (117.4067, 39.3658) -> (117.4067, 37.3658)
  line L565 (117.4067, 42.8658) -> (119.4067, 42.8658)
  line L566 (119.4067, 42.8658) -> (119.4067, 44.8658)
  line L567 (119.4067, 44.8658) -> (117.4067, 44.8658)
  line L568 (117.4067, 44.8658) -> (117.4067, 42.8658)
  line L569 (117.4067, 48.3658) -> (119.4067, 48.3658)
  line L570 (119.4067, 48.3658) -> (119.4067, 50.3658)
  line L571 (119.4067, 50.3658) -> (117.4067, 50.3658)
  line L572 (117.4067, 50.3658) -> (117.4067, 48.3658)
  line L573 (117.4067, 53.8658) -> (119.4067, 53.8658)
  line L574 (119.4067, 53.8658) -> (119.4067, 55.8658)
  line L575 (119.4067, 55.8658) -> (117.4067, 55.8658)
  line L576 (117.4067, 55.8658) -> (117.4067, 53.8658)
  line L577 (117.4067, 59.3658) -> (119.4067, 59.3658)
  line L578 (119.4067, 59.3658) -> (119.4067, 61.3658)
  line L579 (119.4067, 61.3658) -> (117.4067, 61.3658)
  line L580 (117.4067, 61.3658) -> (117.4067, 59.3658)
  line L581 (117.4067, 64.8658) -> (119.4067, 64.8658)
  line L582 (119.4067, 64.8658) -> (119.4067, 66.8658)
  line L583 (119.4067, 66.8658) -> (117.4067, 66.8658)
  line L584 (117.4067, 66.8658) -> (117.4067, 64.8658)
  line L585 (117.4067, 70.3658) -> (119.4067, 70.3658)
  line L586 (119.4067, 70.3658) -> (119.4067, 72.3658)
  line L587 (119.4067, 72.3658) -> (117.4067, 72.3658)
  line L588 (117.4067, 72.3658) -> (117.4067, 70.3658)
  line L589 (121.4067, 37.3658) -> (123.4067, 37.3658)
  line L590 (123.4067, 37.3658) -> (123.4067, 39.3658)
  line L591 (123.4067, 39.3658) -> (121.4067, 39.3658)
  line L592 (121.4067, 39.3658) -> (121.4067, 37.3658)
  line L593 (121.4067, 42.8658) -> (123.4067, 42.8658)
  line L594 (123.4067, 42.8658) -> (123.4067, 44.8658)
  line L595 (123.4067, 44.8658) -> (121.4067, 44.8658)
  line L596 (121.4067, 44.8658) -> (121.4067, 42.8658)
  line L597 (121.4067, 48.3658) -> (123.4067, 48.3658)
  line L598 (123.4067, 48.3658) -> (123.4067, 50.3658)
  line L599 (123.4067, 50.3658) -> (121.4067, 50.3658)
  line L600 (121.4067, 50.3658) -> (121.4067, 48.3658)
  line L601 (121.4067, 53.8658) -> (123.4067, 53.8658)
  line L602 (123.4067, 53.8658) -> (123.4067, 55.8658)
  line L603 (123.4067, 55.8658) -> (121.4067, 55.8658)
  line L604 (121.4067, 55.8658) -> (121.4067, 53.8658)
  line L605 (121.4067, 59.3658) -> (123.4067, 59.3658)
  line L606 (123.4067, 59.3658) -> (123.4067, 61.3658)
  line L607 (123.4067, 61.3658) -> (121.4067, 61.3658)
  line L608 (121.4067, 61.3658) -> (121.4067, 59.3658)
  line L609 (121.4067, 64.8658) -> (123.4067, 64.8658)
  line L610 (123.4067, 64.8658) -> (123.4067, 66.8658)
  line L611 (123.4067, 66.8658) -> (121.4067, 66.8658)
  line L612 (121.4067, 66.8658) -> (121.4067, 64.8658)
  line L613 (121.4067, 70.3658) -> (123.4067, 70.3658)
  line L614 (123.4067, 70.3658) -> (123.4067, 72.3658)
  line L615 (123.4067, 72.3658) -> (121.4067, 72.3658)
  line L616 (121.4067, 72.3658) -> (121.4067, 70.3658)
  line L617 (125.4067, 37.3658) -> (127.4067, 37.3658)
  line L618 (127.4067, 37.3658) -> (127.4067, 39.3658)
  line L619 (127.4067, 39.3658) -> (125.4067, 39.3658)
  line L620 (125.4067, 39.3658) -> (125.4067, 37.3658)
  line L621 (125.4067, 42.8658) -> (127.4067, 42.8658)
  line L622 (127.4067, 42.8658) -> (127.4067, 44.8658)
  line L623 (127.4067, 44.8658) -> (125.4067, 44.8658)
  line L624 (125.4067, 44.8658) -> (125.4067, 42.8658)
  line L625 (125.4067, 48.3658) -> (127.4067, 48.3658)
  line L626 (127.4067, 48.3658) -> (127.4067, 50.3658)
  line L627 (127.4067, 50.3658) -> (125.4067, 50.3658)
  line L628 (125.4067, 50.3658) -> (125.4067, 48.3658)
  line L629 (125.4067, 53.8658) -> (127.4067, 53.8658)
  line L630 (127.4067, 53.8658) -> (127.4067, 55.8658)
  line L631 (127.4067, 55.8658) -> (125.4067, 55.8658)
  line L632 (125.4067, 55.8658) -> (125.4067, 53.8658)
  line L633 (125.4067, 59.3658) -> (127.4067, 59.3658)
  line L634 (127.4067, 59.3658) -> (127.4067, 61.3658)
  line L635 (127.4067, 61.3658) -> (125.4067, 61.3658)
  line L636 (125.4067, 61.3658) -> (125.4067, 59.3658)
  line L637 (125.4067, 64.8658) -> (127.4067, 64.8658)
  line L638 (127.4067, 64.8658) -> (127.4067, 66.8658)
  line L639 (127.4067, 66.8658) -> (125.4067, 66.8658)
  line L640 (125.4067, 66.8658) -> (125.4067, 64.8658)
  line L641 (125.4067, 70.3658) -> (127.4067, 70.3658)
  line L642 (127.4067, 70.3658) -> (127.4067, 72.3658)
  line L643 (127.4067, 72.3658) -> (125.4067, 72.3658)
  line L644 (125.4067, 72.3658) -> (125.4067, 70.3658)
  line L645 (129.4067, 37.3658) -> (131.4067, 37.3658)
  line L646 (131.4067, 37.3658) -> (131.4067, 39.3658)
  line L647 (131.4067, 39.3658) -> (129.4067, 39.3658)
  line L648 (129.4067, 39.3658) -> (129.4067, 37.3658)
  line L649 (129.4067, 42.8658) -> (131.4067, 42.8658)
  line L650 (131.4067, 42.8658) -> (131.4067, 44.8658)
  line L651 (131.4067, 44.8658) -> (129.4067, 44.8658)
  line L652 (129.4067, 44.8658) -> (129.4067, 42.8658)
  line L653 (129.4067, 48.3658) -> (131.4067, 48.3658)
  line L654 (131.4067, 48.3658) -> (131.4067, 50.3658)
  line L655 (131.4067, 50.3658) -> (129.4067, 50.3658)
  line L656 (129.4067, 50.3658) -> (129.4067, 48.3658)
  line L657 (129.4067, 53.8658) -> (131.4067, 53.8658)
  line L658 (131.4067, 53.8658) -> (131.4067, 55.8658)
  line L659 (131.4067, 55.8658) -> (129.4067, 55.8658)
  line L660 (129.4067, 55.8658) -> (129.4067, 53.8658)
  line L661 (129.4067, 59.3658) -> (131.4067, 59.3658)
  line L662 (131.4067, 59.3658) -> (131.4067, 61.3658)
  line L663 (131.4067, 61.3658) -> (129.4067, 61.3658)
  line L664 (129.4067, 61.3658) -> (129.4067, 59.3658)
  line L665 (129.4067, 64.8658) -> (131.4067, 64.8658)
  line L666 (131.4067, 64.8658) -> (131.4067, 66.8658)
  line L667 (131.4067, 66.8658) -> (129.4067, 66.8658)
  line L668 (129.4067, 66.8658) -> (129.4067, 64.8658)
  line L669 (129.4067, 70.3658) -> (131.4067, 70.3658)
  line L670 (131.4067, 70.3658) -> (131.4067, 72.3658)
  line L671 (131.4067, 72.3658) -> (129.4067, 72.3658)
  line L672 (129.4067, 72.3658) -> (129.4067, 70.3658)
  line L673 (35.4067, 39.3658) -> (35.4067, 37.3658) projected
  point P0 (0, 0)
  point P1 (37.4067, 38.3658)
  point P2 (37.4067, 43.8658)
  point P3 (37.4067, 49.3658)
  point P4 (37.4067, 54.8658)
  point P5 (37.4067, 60.3658)
  point P6 (37.4067, 65.8658)
  point P7 (37.4067, 71.3658)
  point P8 (41.4067, 38.3658)
  point P9 (41.4067, 43.8658)
  point P10 (41.4067, 49.3658)
  point P11 (41.4067, 54.8658)
  point P12 (41.4067, 60.3658)
  point P13 (41.4067, 65.8658)
  point P14 (41.4067, 71.3658)
  point P15 (45.4067, 38.3658)
  point P16 (45.4067, 43.8658)
  point P17 (45.4067, 49.3658)
  point P18 (45.4067, 54.8658)
  point P19 (45.4067, 60.3658)
  point P20 (45.4067, 65.8658)
  point P21 (45.4067, 71.3658)
  point P22 (49.4067, 38.3658)
  point P23 (49.4067, 43.8658)
  point P24 (49.4067, 49.3658)
  point P25 (49.4067, 54.8658)
  point P26 (49.4067, 60.3658)
  point P27 (49.4067, 65.8658)
  point P28 (49.4067, 71.3658)
  point P29 (53.4067, 38.3658)
  point P30 (53.4067, 43.8658)
  point P31 (53.4067, 49.3658)
  point P32 (53.4067, 54.8658)
  point P33 (53.4067, 60.3658)
  point P34 (53.4067, 65.8658)
  point P35 (53.4067, 71.3658)
  point P36 (57.4067, 38.3658)
  point P37 (57.4067, 43.8658)
  point P38 (57.4067, 49.3658)
  point P39 (57.4067, 54.8658)
  point P40 (57.4067, 60.3658)
  point P41 (57.4067, 65.8658)
  point P42 (57.4067, 71.3658)
  point P43 (61.4067, 38.3658)
  point P44 (61.4067, 43.8658)
  point P45 (61.4067, 49.3658)
  point P46 (61.4067, 54.8658)
  point P47 (61.4067, 60.3658)
  point P48 (61.4067, 65.8658)
  point P49 (61.4067, 71.3658)
  point P50 (65.4067, 38.3658)
  point P51 (65.4067, 43.8658)
  point P52 (65.4067, 49.3658)
  point P53 (65.4067, 54.8658)
  point P54 (65.4067, 60.3658)
  point P55 (65.4067, 65.8658)
  point P56 (65.4067, 71.3658)
  point P57 (69.4067, 38.3658)
  point P58 (69.4067, 43.8658)
  point P59 (69.4067, 49.3658)
  point P60 (69.4067, 54.8658)
  point P61 (69.4067, 60.3658)
  point P62 (69.4067, 65.8658)
  point P63 (69.4067, 71.3658)
  point P64 (73.4067, 38.3658)
  point P65 (73.4067, 43.8658)
  point P66 (73.4067, 49.3658)
  point P67 (73.4067, 54.8658)
  point P68 (73.4067, 60.3658)
  point P69 (73.4067, 65.8658)
  point P70 (73.4067, 71.3658)
  point P71 (77.4067, 38.3658)
  point P72 (77.4067, 43.8658)
  point P73 (77.4067, 49.3658)
  point P74 (77.4067, 54.8658)
  point P75 (77.4067, 60.3658)
  point P76 (77.4067, 65.8658)
  point P77 (77.4067, 71.3658)
  point P78 (81.4067, 38.3658)
  point P79 (81.4067, 43.8658)
  point P80 (81.4067, 49.3658)
  point P81 (81.4067, 54.8658)
  point P82 (81.4067, 60.3658)
  point P83 (81.4067, 65.8658)
  point P84 (81.4067, 71.3658)
  point P85 (85.4067, 38.3658)
  point P86 (85.4067, 43.8658)
  point P87 (85.4067, 49.3658)
  point P88 (85.4067, 54.8658)
  point P89 (85.4067, 60.3658)
  point P90 (85.4067, 65.8658)
  point P91 (85.4067, 71.3658)
  point P92 (89.4067, 38.3658)
  point P93 (89.4067, 43.8658)
  point P94 (89.4067, 49.3658)
  point P95 (89.4067, 54.8658)
  point P96 (89.4067, 60.3658)
  point P97 (89.4067, 65.8658)
  point P98 (89.4067, 71.3658)
  point P99 (93.4067, 38.3658)
  point P100 (93.4067, 43.8658)
  point P101 (93.4067, 49.3658)
  point P102 (93.4067, 54.8658)
  point P103 (93.4067, 60.3658)
  point P104 (93.4067, 65.8658)
  point P105 (93.4067, 71.3658)
  point P106 (97.4067, 38.3658)
  point P107 (97.4067, 43.8658)
  point P108 (97.4067, 49.3658)
  point P109 (97.4067, 54.8658)
  point P110 (97.4067, 60.3658)
  point P111 (97.4067, 65.8658)
  point P112 (97.4067, 71.3658)
  point P113 (101.4067, 38.3658)
  point P114 (101.4067, 43.8658)
  point P115 (101.4067, 49.3658)
  point P116 (101.4067, 54.8658)
  point P117 (101.4067, 60.3658)
  point P118 (101.4067, 65.8658)
  point P119 (101.4067, 71.3658)
  point P120 (105.4067, 38.3658)
  point P121 (105.4067, 43.8658)
  point P122 (105.4067, 49.3658)
  point P123 (105.4067, 54.8658)
  point P124 (105.4067, 60.3658)
  point P125 (105.4067, 65.8658)
  point P126 (105.4067, 71.3658)
  point P127 (109.4067, 38.3658)
  point P128 (109.4067, 43.8658)
  point P129 (109.4067, 49.3658)
  point P130 (109.4067, 54.8658)
  point P131 (109.4067, 60.3658)
  point P132 (109.4067, 65.8658)
  point P133 (109.4067, 71.3658)
  point P134 (113.4067, 38.3658)
  point P135 (113.4067, 43.8658)
  point P136 (113.4067, 49.3658)
  point P137 (113.4067, 54.8658)
  point P138 (113.4067, 60.3658)
  point P139 (113.4067, 65.8658)
  point P140 (113.4067, 71.3658)
  point P141 (117.4067, 38.3658)
  point P142 (117.4067, 43.8658)
  point P143 (117.4067, 49.3658)
  point P144 (117.4067, 54.8658)
  point P145 (117.4067, 60.3658)
  point P146 (117.4067, 65.8658)
  point P147 (117.4067, 71.3658)
  point P148 (121.4067, 38.3658)
  point P149 (121.4067, 43.8658)
  point P150 (121.4067, 49.3658)
  point P151 (121.4067, 54.8658)
  point P152 (121.4067, 60.3658)
  point P153 (121.4067, 65.8658)
  point P154 (121.4067, 71.3658)
  point P155 (125.4067, 38.3658)
  point P156 (125.4067, 43.8658)
  point P157 (125.4067, 49.3658)
  point P158 (125.4067, 54.8658)
  point P159 (125.4067, 60.3658)
  point P160 (125.4067, 65.8658)
  point P161 (125.4067, 71.3658)
  point P162 (129.4067, 38.3658)
  point P163 (129.4067, 43.8658)
  point P164 (129.4067, 49.3658)
  point P165 (129.4067, 54.8658)
  point P166 (129.4067, 60.3658)
  point P167 (129.4067, 65.8658)
  point P168 (129.4067, 71.3658)
  dimension "d111" = 2
  dimension "d112" = 2
  dimension "d113" = 1
  dimension "d116" = 5.5
  dimension "d119" = 4
  dimension "d124" = 2
  constraints: 1344 end point, 2 collinear, 2 horizontal, 2 parallel, 1 midpoint, 1 perpendicular, 1 vertical, 1501 other
  measures "d111" distance of L0.start L0.end
  measures "d112" distance of L0.end L1.end
  measures "d113" distance from line of L4 point (37.407, 38.366)
  measures "d116" distance of L0.start L5.start
  measures "d119" distance of L0.start L29.start
  measures "d124" distance between parallel lines of L3 L673
extrude "Extrusion8" cut sketch "Sketch12" against normal blind 10
body "Solid1"
